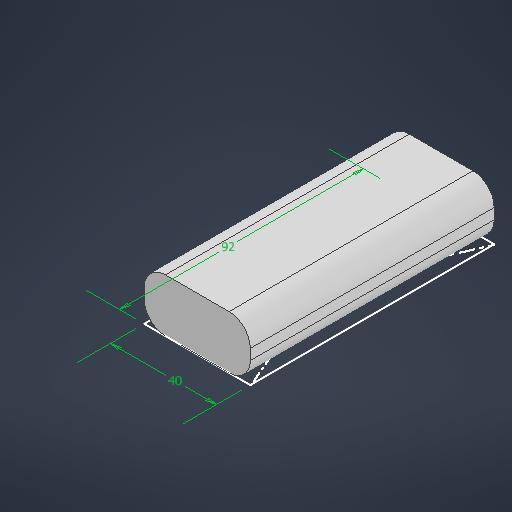
# Autodesk Inventor part: battery-model-group2
Saved by Autodesk Inventor 2026.1 (Build 301233000, 233)
## iProperties
Created: 2026-02-24
Part Number: battery-model-group2
Material: Generic
Document SubType Name: Modeling
Designer: aj2074
Density: 1 g/cm^3
Appearance: Default
Author: aj2074
Autodesk Inventor part; units mm, degrees
ref_plane "YZ Plane" through (0, 0, 0) normal (1, 0, 0) x (0, 1, 0)
ref_plane "XZ Plane" through (0, 0, 0) normal (0, 1, 0) x (-1, 0, 0)
ref_plane "XY Plane" through (0, 0, 0) normal (0, 0, 1) x (1, 0, 0)
sketch "Sketch1" plane through (0, 0, 0) normal (0, 1, 0) x (-1, 0, 0)
  line L0 (20, 46) -> (-20, 46)
  line L1 (-20, 46) -> (-20, -46)
  line L2 (-20, -46) -> (20, -46)
  line L3 (20, -46) -> (20, 46)
  line L4 (20, 46) -> (-20, -46)
  line L5 (20, -46) -> (-20, 46)
  point P0 (0, 0)
  point P1 (0, 0)
  dimension "d9" = 92
  dimension "d10" = 40
  constraints: 12 end point, 2 midpoint, 2 parallel, 1 coincident, 1 horizontal, 1 perpendicular
  measures "d9" distance of L2.end L0.start
  measures "d10" distance between parallel lines of L1 L3
extrude "Extrusion1" add sketch "Sketch1" along normal blind 20
fillet "Fillet5" radius 8 4 edges at (20, 20, 0) (-20, 20, 0) (20, 0, 0) (-20, 0, 0)
